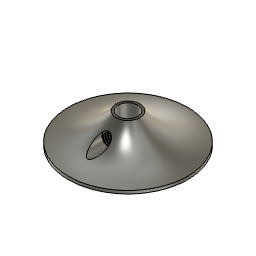
1_4 Rod Foot v3 (Autodesk Fusion 360 design; units mm, degrees)
Autodesk Fusion 360 part; units mm, degrees
sketch "Sketch1" plane through (0, 0, 0) normal (0, 0, 1) x (1, 0, 0)
  circle A0 centre (0, 0) radius 3.3
  circle A1 centre (0, 0) radius 20
  dimension "d1" = 6.6
  constraint coincident A0.centre A1.centre
  measures "d1" diameter of A0
sketch "Sketch2" plane through (0, 0, 0) normal (0, 1, 0) x (1, 0, 0)
  line L0 (20, 0) -> (3.3, 0)
  line L1 (3.3, 0) -> (3.3, -10)
  arc A0 (20, -1) -> (4, -10) centre (23.0455, -25.1364) ccw
  line L2 (3.3, -10) -> (4, -10)
  line L3 (20, -1) -> (20, 0)
  line L4 (4, -10) -> (20, -10)
  line L5 (20, -10) -> (20, -1)
  constraint horizontal L0
  constraint perpendicular L0 L1
  constraint perpendicular L1 L2
  constraint perpendicular L2 L3
  constraint parallel L2 L4
  constraint perpendicular L4 L5
revolve "Revolve1" add sketch "Sketch2" angle 360 about axis through (0, 0, 1.75) along (0, 0, 1) contours L0 L1 A0 L2 L3 makes body 1
sketch "Sketch3" plane through (0, 0, 0) normal (0, 1, 0) x (1, 0, 0)
  circle A0 centre (0, -5) radius 0.5
  circle A1 centre (0, -5) radius 2
  circle A2 centre (0, -5) radius 2.25
  dimension "d5" = 4.5
  constraint concentric A0 A1
  constraint concentric A1 A2
  measures "d5" diameter of A2
extrude "Extrude1" add sketch "Sketch3" against normal blind 15 contours A0 | A1 bodies 1
extrude "Extrude2" add sketch "Sketch3" against normal blind 15 contours A2 bodies 1
hole "Hole1" at (0, -15, 5) direction (0, 1, 0) diameter 3.416 depth 16 tip angle 180 bodies 1
thread "Thread1" "ANSI Unified Screw Threads 0.164(#8) 8-32 UNC 2B" major diameter 4.1656 minor diameter 3.4163 pitch 0.7937 angle 60 modelled right hand crest width 0.2341 on face at (0.1701, -10, 3.3005) crest through (0, -14.8016, 3.2919) on bodies 1
extrude "Extrude3" cut sketch "Sketch3" against normal blind 3.5 contours A1 | A2 bodies 1
extrude "Extrude4" cut sketch "Sketch3" against normal blind 11 from surface at -7.5 contours A1 | A2 bodies 1
revolve "Revolve2" cut sketch "Sketch2" angle 360 about axis through (0, 0, 1.75) along (0, 0, 1) contours A0 L4 L5 bodies 1
extrude "Extrude5" cut sketch "Sketch3" against normal blind 9.5 from surface at -6.5 contours A1 | A2 bodies 1
sketch "Sketch1 (2)" plane through (0, 0, 0) normal (0, 0, 1) x (1, 0, 0) in component "4 Rod Base"
  line L0 (0, 0) -> (21.2132, 21.2132)
  line L1 (0, 0) -> (30, 0) construction
  line L2 (0, 0) -> (-21.2132, 21.2132)
  line L3 (0, 0) -> (-21.2132, -21.2132)
  line L4 (0, 0) -> (21.2132, -21.2132)
  circle A0 centre (-21.2132, 21.2132) radius 3.3
  circle A1 centre (-21.2132, -21.2132) radius 3.3
  circle A2 centre (21.2132, 21.2132) radius 3.3
  circle A3 centre (21.2132, -21.2132) radius 3.3
  line L5 (37.5, -37.5) -> (-37.5, -37.5)
  line L6 (-37.5, -37.5) -> (-37.5, 37.5)
  line L7 (-37.5, 37.5) -> (37.5, 37.5)
  line L8 (37.5, 37.5) -> (37.5, -37.5)
  line L9 (37.5, -37.5) -> (-37.5, 37.5) construction
  line L10 (-37.5, -37.5) -> (37.5, 37.5) construction
  dimension "d20" = 30
  dimension "d21" = 45
  dimension "d22" = 30
  dimension "d23" = 30
  dimension "d24" = 30
  dimension "d25" = 6.6
  dimension "d26" = 6.6
  dimension "d27" = 6.6
  dimension "d28" = 6.6
  dimension "d29" = 75
  dimension "d30" = 75
  constraint horizontal L1
  constraint coincident L0.start L1.start
  constraint perpendicular L0 L2
  constraint perpendicular L2 L3
  constraint perpendicular L3 L4
  constraint coincident L2.end A0.centre
  constraint coincident L3.end A1.centre
  constraint coincident L0.end A2.centre
  constraint coincident L4.end A3.centre
  constraint horizontal L5
  constraint perpendicular L5 L6
  constraint parallel L5 L7
  constraint parallel L6 L8
  constraint coincident L9 L0.start
  constraint coincident L10 L0.start
  measures "d20" distance of L0.start L0.end
  measures "d21" angle of L0 L1
  measures "d22" distance of L0.start L2.end
  measures "d23" distance of L0.start L3.end
  measures "d24" distance of L0.start L4.end
  measures "d25" diameter of A0
  measures "d26" diameter of A1
  measures "d27" diameter of A2
  measures "d28" diameter of A3
  measures "d29" distance of L6.end L7.end
  measures "d30" distance of L5.end L6.end
sketch "Sketch1 (3)" plane through (0, 0, 0) normal (0, 0, 1) x (1, 0, 0) in component "2 Rod Base"
  line L0 (0, 0) -> (-21.2132, 21.2132)
  line L1 (0, 0) -> (21.2132, 21.2132)
  circle A0 centre (21.2132, 21.2132) radius 3.3
  circle A1 centre (-21.2132, 21.2132) radius 3.3
  line L2 (-21.2132, 21.2132) -> (21.2132, 21.2132)
  line L3 (0, 21.2132) -> (0, 0)
  line L4 (40, 1.2132) -> (-40, 1.2132)
  line L5 (-40, 1.2132) -> (-40, 41.2132)
  line L6 (-40, 41.2132) -> (40, 41.2132)
  line L7 (40, 41.2132) -> (40, 1.2132)
  line L8 (40, 1.2132) -> (-40, 41.2132) construction
  line L9 (-40, 1.2132) -> (40, 41.2132) construction
  point P0 (0, 21.2132)
  dimension "d31" = 30
  dimension "d32" = 30
  dimension "d33" = 6.6
  dimension "d34" = 6.6
  dimension "d35" = 40
  constraint coincident L0.start L1.start
  constraint perpendicular L0 L1
  constraint coincident L1.end A0.centre
  constraint coincident L0.end A1.centre
  constraint horizontal L2
  constraint midpoint L2 P0
  constraint horizontal L4
  constraint perpendicular L4 L5
  constraint parallel L4 L6
  constraint parallel L5 L7
  constraint coincident L8 P0
  constraint coincident L9 P0
  constraint coincident P0 L3.start
  measures "d31" distance of L0.start L0.end
  measures "d32" distance of L0.start L1.end
  measures "d33" diameter of A0
  measures "d34" diameter of A1
  measures "d35" distance of L4.end L5.end
extrude "Extrude1'" add sketch "Sketch1 (3)" along normal blind 5 separate body contours L0 L1 A0 A1 L2 L4 L5 L6 L7 | L0 A1 L2 L3 L4 | L1 A0 L2 L3 L4 makes body 2 in component "2 Rod Base"
component "4 Rod Base" placed x (1, 0, 0) y (0, 1, 0) z (0, 0, 1) at (0, 0, 0)
component "2 Rod Base" placed x (1, 0, 0) y (0, 1, 0) z (0, 0, 1) at (0, 0, 0) in component "4 Rod Base"
named bodies: "1/4 Rod Foot"
